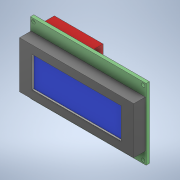
# Autodesk Inventor part: LcdAssembly
Saved by Autodesk Inventor 2020 (Build 240168000, 168)
## iProperties
Created: 2019-12-15
Part Number: LcdAssembly
Material: Generic
Document SubType Name: Modeling
Designer: torto
Density: 1 g/cm^3
Appearance: Default
Author: torto
Autodesk Inventor part; units mm, degrees
ref_plane "YZ Plane" through (0, 0, 0) normal (1, 0, 0) x (0, 1, 0)
ref_plane "XZ Plane" through (0, 0, 0) normal (0, 1, 0) x (-1, 0, 0)
ref_plane "XY Plane" through (0, 0, 0) normal (0, 0, 1) x (1, 0, 0)
sketch "Sketch1" plane through (0, 0, 0) normal (0, 0, 1) x (1, 0, 0)
  line L0 (0, 0) -> (98.25, 0)
  line L1 (98.25, 0) -> (98.25, 60.25)
  line L2 (98.25, 60.25) -> (0, 60.25)
  line L3 (0, 60.25) -> (0, 0)
  line L4 (0, 60.25) -> (2.5, 60.25) construction
  line L5 (2.5, 60.25) -> (2.5, 57.75) construction
  line L6 (2.5, 57.75) -> (0, 57.75) construction
  line L7 (0, 57.75) -> (0, 60.25) construction
  circle A0 centre (2.5, 57.75) radius 1.5
  line L8 (49.125, 60.25) -> (49.125, 0) construction
  line L9 (0, 30.125) -> (98.25, 30.125) construction
  circle A1 centre (95.75, 57.75) radius 1.5
  circle A2 centre (2.5, 2.5) radius 1.5
  circle A3 centre (95.75, 2.5) radius 1.5
  dimension "d0" = 98.25
  dimension "d1" = 60.25
  dimension "d2" = 2.5
  dimension "d7" = 2.5
  dimension "d8" = 3
  constraints: 20 end point, 4 centre point, 4 midpoint, 4 parallel, 3 symmetric about line, 2 horizontal, 2 perpendicular, 1 coincident, 3 other
  measures "d0" distance of L1.end L2.end
  measures "d1" distance of L0.end L1.end
  measures "d2" distance of L4.end L5.end
  measures "d7" distance of L5.end L6.end
  measures "d8" diameter of A0
extrude "LcdPcb" add sketch "Sketch1" along normal blind 2.8
sketch "Sketch2" plane through (0, 0, 2.8) normal (0, 0, 1) x (1, 0, 0)
  line L0 (98.25, 60.25) -> (0, 60.25) construction
  line L1 (49.125, 60.25) -> (49.125, 0) construction
  line L2 (0, 0) -> (98.25, 0) construction
  line L3 (0, 60.25) -> (0, 0) construction
  line L4 (0, 30.125) -> (98.25, 30.125) construction
  line L5 (98.25, 0) -> (98.25, 60.25) construction
  line L6 (0.575, 50.025) -> (97.675, 50.025)
  line L7 (97.675, 50.025) -> (97.675, 10.225)
  line L8 (97.675, 10.225) -> (0.575, 10.225)
  line L9 (0.575, 10.225) -> (0.575, 50.025)
  line L10 (0.575, 50.025) -> (97.675, 10.225) construction
  line L11 (97.675, 50.025) -> (0.575, 10.225) construction
  point P0 (49.125, 30.125)
  dimension "d15" = 39.8
  dimension "d16" = 97.1
  constraints: 16 end point, 7 midpoint, 2 parallel, 1 horizontal, 1 perpendicular
  measures "d15" distance of L6.end L7.end
  measures "d16" distance of L7.end L8.end
extrude "LcdBezel" add sketch "Sketch2" along normal blind 9.9
sketch "Sketch3" plane through (0, 0, 12.7) normal (0, 0, 1) x (1, 0, 0)
  line L0 (0.575, 50.025) -> (0.575, 10.225) construction
  line L1 (0.575, 50.025) -> (11.375, 50.025) construction
  line L2 (11.375, 50.025) -> (11.375, 43.125) construction
  line L3 (11.375, 43.125) -> (0.575, 43.125) construction
  line L4 (0.575, 43.125) -> (0.575, 50.025) construction
  line L5 (11.375, 43.125) -> (86.875, 43.125)
  line L6 (86.875, 43.125) -> (86.875, 17.125)
  line L7 (86.875, 17.125) -> (11.375, 17.125)
  line L8 (11.375, 17.125) -> (11.375, 43.125)
  point P0 (0, 0)
  dimension "LcdBezelHeight" = 6.9
  dimension "LcdBezelLength" = 10.8
  dimension "d28" = 75.5
  dimension "d29" = 26
  constraints: 16 end point, 4 parallel, 2 horizontal, 2 perpendicular
  measures "LcdBezelHeight" distance of L1.end L2.end
  measures "LcdBezelLength" distance of L2.end L3.end
  measures "d28" distance of L6.end L7.end
  measures "d29" distance of L5.end L6.end
extrude "Lcd" cut sketch "Sketch3" against normal blind 1.4
sketch "Sketch4" plane through (0, 0, 0) normal (0, 0, -1) x (-1, 0, 0)
  line L0 (0, 60.25) -> (0, 0) construction
  line L1 (0, 60.25) -> (-7.5, 60.25) construction
  line L2 (-7.5, 60.25) -> (-7.5, 58.25) construction
  line L3 (-7.5, 58.25) -> (0, 58.25) construction
  line L4 (0, 58.25) -> (0, 60.25) construction
  line L5 (-7.5, 58.25) -> (-49, 58.25)
  line L6 (-49, 58.25) -> (-49, 39.25)
  line L7 (-49, 39.25) -> (-7.5, 39.25)
  line L8 (-7.5, 39.25) -> (-7.5, 58.25)
  dimension "LcdRearKeepOutHeightOffset" = 2
  dimension "LcdRearKeepOutLengthOffset" = 7.5
  dimension "LcdRearKeepOutHeight" = 19
  dimension "LcdRearKeepOutLength" = 41.5
  constraints: 16 end point, 4 parallel, 2 horizontal, 2 perpendicular
  measures "LcdRearKeepOutHeightOffset" distance of L1.end L2.end
  measures "LcdRearKeepOutLengthOffset" distance of L2.end L3.end
  measures "LcdRearKeepOutHeight" distance of L5.end L6.end
  measures "LcdRearKeepOutLength" distance of L6.end L7.end
extrude "LcdRearKeepOut" add sketch "Sketch4" along normal blind 10
equation "\"d0\" = LcdBorderLength"
equation "\"d1\" = LcdBorderHeight"
equation "\"d2\" = LcdFrameHoleOffset"
equation "\"d7\" = LcdFrameHoleOffset"
equation "\"d8\" = LcdFrameHoleDiameter"
equation "\"d12\" = LcdPcbThickness"
equation "\"d15\" = LcdHeight"
equation "\"d16\" = LcdLength"
equation "\"d28\" = LcdLength - 2 * LcdBezelLength"
equation "\"d29\" = LcdHeight - 2 * LcdBezelHeight"
equation "\"d30\" = 0.5 * LcdPcbThickness"
equation "\"LcdBorderLength\" = 98.25"
equation "\"LcdBorderHeight\" = 60.25"
equation "\"LcdFrameHoleOffset\" = 2.5"
equation "\"LcdFrameHoleDiameter\" = 3"
equation "\"LcdPcbThickness\" = 2.8"
equation "\"LcdHeight\" = 39.8"
equation "\"LcdLength\" = 97.1"
body "Solid1"
